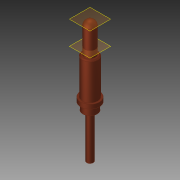
# Autodesk Inventor part: Federkontakt D1.5
Saved by Autodesk Inventor 2019.3 (Build 233278000, 278)
## iProperties
Part Number: Federkontakt D1.5
Material: Kupfer, Legierung
Document SubType Name: Modeling
Designer: rYan
Mass: 0.0923712 g
Surface Area: 0.331014 cm^2
Volume: 0.0103555 cm^3
Density: 8.92 g/cm^3
Appearance: Kupfer - satiniert
Title: 0928-0-15-20-77-14-11-0
Author: rYan
Autodesk Inventor part; units mm, degrees
ref_plane "YZ Plane" through (0, 0, 0) normal (1, 0, 0) x (0, 1, 0)
ref_plane "XZ Plane" through (0, 0, 0) normal (0, 1, 0) x (-1, 0, 0)
sketch "Skizze1" plane through (0, 0, 0) normal (0, 1, 0) x (-1, 0, 0)
  line L0 (0, -5.01) -> (0, 6.96)
  line L1 (-0.7, 0) -> (-0.915, 0)
  line L2 (-0.915, 0) -> (-0.915, 0.41)
  line L3 (-0.915, 0.41) -> (-0.75, 0.41)
  line L4 (-0.75, 0.41) -> (-0.75, 3.99)
  line L5 (-0.75, 3.99) -> (-0.535, 3.99)
  line L6 (-0.535, 3.99) -> (-0.535, 6.425)
  arc A0 (0, 6.96) -> (-0.535, 6.425) centre (0, 6.425) ccw
  line L7 (-0.535, 6.425) -> (0, 6.425) construction
  line L8 (-0.7, 0) -> (-0.7, -0.71)
  line L9 (-0.7, -0.71) -> (-0.32, -0.71)
  line L10 (-0.32, -0.71) -> (-0.32, -5.01)
  line L11 (-0.32, -5.01) -> (0, -5.01)
  line L12 (0, -7.4262) -> (0, 9.487) projected
  line L13 (-1.098, 0) -> (0.183, 0) projected
  dimension "d0" = 1.07
  dimension "d1" = 0.41
  dimension "d2" = 1.83
  dimension "d3" = 1.5
  dimension "d5" = 6.96
  dimension "d10" = 0.71
  dimension "d11" = 0.7
  dimension "d12" = 4.3
  dimension "d15" = 0.64
  dimension "d16" = 4.7
  constraints: 24 end point, 9 perpendicular, 2 point on circle, 2 point on line, 2 vertical, 1 centre point, 1 collinear, 1 horizontal
  measures "d0" diameter of L6 L0
  measures "d1" distance of L1.end L2.end
  measures "d2" diameter of L2 L0
  measures "d3" diameter of L4 L0
  measures "d5" distance from line of L1 L0.end
  measures "d10" distance of L1.start L8.end
  measures "d11" distance between parallel lines of L12 L8
  measures "d12" distance of L9.end L10.end
  measures "d15" diameter of L10 L0
  measures "d16" distance between parallel lines of L5 L9
revolve "Umdrehung1" add sketch "Skizze1" angle 360 about axis through (0, 0, -5.01) along (0, 0, 1)
chamfer "Fase1" distance 0.1 angle 45 1 edges at (-0.75, 0, 3.99)
ref_plane "Arbeitsebene2" through (0, 0, 4.67) normal (0, 0, 1) x (1, 0, 0)
ref_plane "Arbeitsebene1" through (0, 0, 6.96) normal (0, 0, 1) x (1, 0, 0)
